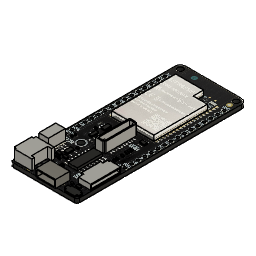
Wemos D32 Pro v13 (Autodesk Fusion 360 design; units mm, degrees)
Autodesk Fusion 360 part; units mm, degrees
sketch "Skizze1" plane through (0, 0, 0) normal (0, 0, 1) x (1, 0, 0)
  line L0 (-12.7, 32.5) -> (12.7, 32.5)
  line L1 (12.7, 32.5) -> (12.7, -32.5)
  line L2 (12.7, -32.5) -> (-12.7, -32.5)
  line L3 (-12.7, -32.5) -> (-12.7, 32.5)
  line L4 (0, 32.5) -> (0, -32.5)
  line L5 (12.7, 0) -> (-12.7, 0)
  line L6 (-8.0924, -22.0419) -> (-2.6557, -22.0419)
  line L7 (-2.6557, -22.0419) -> (-2.6557, -26)
  dimension "d1" = 65
  dimension "d2" = 25.4
  constraint horizontal L0
  constraint vertical L1
  constraint horizontal L2
  constraint vertical L3
  constraint midpoint L0 L4.start
  constraint midpoint L2 L4.end
  constraint coincident origin L4
  constraint midpoint L1 L5.start
  constraint midpoint L3 L5.end
  constraint coincident origin L5
  measures "d1" distance of L0 L2
  measures "d2" distance of L1 L3
extrude "Extrusion1" add sketch "Skizze1" along normal blind 1.57 makes body 1
fillet "Abrundung1" radius 1 2 edges at (12.7, -32.5, 0.785) (-12.7, -32.5, 0.785) on bodies 1
fillet "Abrundung2" radius 2 2 edges at (12.7, 32.5, 0.785) (-12.7, 32.5, 0.785) on bodies 1
sketch "Skizze2" plane through (0, 0, 1.57) normal (0, 0, 1) x (-1, 0, 0)
  arc A0 (10.7, -32.5) -> (12.7, -30.5) centre (10.7, -30.5) ccw
  line L0 (12.7, -30.5) -> (12.7, 31.5)
  arc A1 (12.7, 31.5) -> (11.7, 32.5) centre (11.7, 31.5) ccw
  line L1 (11.7, 32.5) -> (-11.7, 32.5)
  arc A2 (-11.7, 32.5) -> (-12.7, 31.5) centre (-11.7, 31.5) ccw
  line L2 (-12.7, 31.5) -> (-12.7, -30.5)
  arc A3 (-12.7, -30.5) -> (-10.7, -32.5) centre (-10.7, -30.5) ccw
  line L3 (-10.7, -32.5) -> (10.7, -32.5)
  circle A4 centre (5.3, 12.9) radius 1.1365
  circle A5 centre (-11.4, 12.8) radius 0.5
  point P0 (10.7, -30.5)
  point P1 (-10.7, -30.5)
  dimension "d29" = 1
  constraint coincident P0 A0.centre
  constraint coincident P1 A3.centre
  measures "d29" diameter of A5
hole "Bohrung1" at (-10.7, 30.5, 1.57) at (10.7, 30.5, 1.57) direction (0, 0, -1) diameter 2.1 end through all bodies 1
extrude "Extrusion2" cut sketch "Skizze2" against normal through all contours A4 bodies 1
sketch "Skizze3" plane through (0, 0, 1.57) normal (0, 0, 1) x (-1, 0, 0)
  circle A0 centre (5.3, 12.9) radius 1.1365
  circle A1 centre (10.7, -30.5) radius 1.05
  circle A2 centre (-10.7, -30.5) radius 1.05
  arc A3 (10.7, -32.5) -> (12.7, -30.5) centre (10.7, -30.5) ccw
  line L0 (12.7, -30.5) -> (12.7, 31.5)
  arc A4 (12.7, 31.5) -> (11.7, 32.5) centre (11.7, 31.5) ccw
  line L1 (11.7, 32.5) -> (-11.7, 32.5)
  arc A5 (-11.7, 32.5) -> (-12.7, 31.5) centre (-11.7, 31.5) ccw
  line L2 (-12.7, 31.5) -> (-12.7, -30.5)
  arc A6 (-12.7, -30.5) -> (-10.7, -32.5) centre (-10.7, -30.5) ccw
  line L3 (-10.7, -32.5) -> (10.7, -32.5)
  line L4 (8, -26) -> (-8.0924, -26)
  line L5 (-8.0924, -26) -> (-8.0924, -1.543)
  line L6 (-8.0924, -1.543) -> (8, -1.543)
  line L7 (8, -1.543) -> (8, -26)
  line L8 (-8.0924, -22.0419) -> (-2.6557, -22.0419)
  line L9 (-2.6557, -22.0419) -> (-2.6557, -26)
  line L10 (0.3, 12.3) -> (-2.4695, 12.3)
  line L11 (-3.0004, 11.7003) -> (-3.0073, 0.1927)
  line L12 (-3.0073, 0.1927) -> (-2.6232, 0.1927)
  line L13 (-2.6232, 0.1927) -> (-2.6232, -0.5)
  line L14 (-2.6232, -0.5) -> (0.1, -0.5)
  line L15 (0.1, -0.5) -> (0.3, 12.3)
  line L16 (-2.4695, 12.3) -> (-2.4695, 11.7)
  line L17 (-2.4695, 11.7) -> (-3.0004, 11.7003)
  line L18 (12.7, 31.017) -> (12, 31.017)
  line L19 (12, 31.017) -> (12, 31.7213)
  line L20 (12, 31.7213) -> (5.2889, 31.7213)
  line L21 (5.2889, 31.7213) -> (5.2889, 30.6934)
  line L22 (5.2889, 30.6934) -> (6.5, 30.6934)
  line L23 (6.5, 30.6934) -> (6.5, 24.5)
  line L24 (6.5, 24.5) -> (5, 24.5)
  line L25 (5, 24.5) -> (5, 23.5)
  line L26 (5, 23.5) -> (11.9879, 23.5)
  line L27 (11.9879, 23.5) -> (11.9879, 24.4)
  line L28 (11.9879, 24.4) -> (12.7, 24.4)
  line L29 (2.5, 27.5) -> (-5, 27.5)
  line L30 (-5, 27.5) -> (-5, 33)
  line L31 (-5, 33) -> (2.5, 33)
  line L32 (2.5, 33) -> (2.5, 27.5)
  line L33 (-12.284, 15.3134) -> (-8.2222, 15.3134)
  line L34 (-8.2222, 15.3134) -> (-8.2222, 15.7057)
  line L35 (-8.2222, 15.7057) -> (-7.6, 15.7057)
  line L36 (-7.6, 15.7057) -> (-7.6, 17.4)
  line L37 (-7.6, 17.4) -> (-6.7, 17.4)
  line L38 (-6.7, 17.4) -> (-6.7, 24.7236)
  line L39 (-6.7, 24.7236) -> (-7.6, 24.7236)
  line L40 (-7.6, 24.7236) -> (-7.6, 26.8499)
  line L41 (-7.6, 26.8499) -> (-12.2869, 26.8499)
  line L42 (-12.2869, 26.8499) -> (-12.284, 15.3134)
  line L43 (0.2178, 13.2376) -> (-3.3, 13.2376)
  line L44 (-3.3, 13.2376) -> (-3.3, 23)
  line L45 (-3.3, 23) -> (0.2178, 23)
  line L46 (0.2178, 23) -> (0.2178, 13.2376)
  line L47 (-7.6661, 29.4452) -> (-11.5851, 29.4452)
  line L48 (-11.5851, 29.4452) -> (-11.5851, 32.3121)
  line L49 (-11.5851, 32.3121) -> (-7.6661, 32.3121)
  line L50 (-7.6661, 32.3121) -> (-7.6661, 29.4452)
  line L51 (-6.7206, 29.9485) -> (-7.6661, 29.9485)
  line L52 (-7.6661, 29.9485) -> (-7.6661, 31.3971)
  line L53 (-7.6661, 31.3971) -> (-6.7206, 31.3971)
  line L54 (-6.7206, 31.3971) -> (-6.7206, 29.9485)
  line L55 (-11.5851, 30.0095) -> (-12.3019, 30.0095)
  line L56 (-12.3019, 30.0095) -> (-12.3019, 31.3971)
  line L57 (-12.3019, 31.3971) -> (-11.5851, 31.3971)
  line L58 (-11.5851, 31.3971) -> (-11.5851, 30.0095)
  line L59 (-8.3371, 27.7983) -> (-9.9382, 27.7983)
  line L60 (-9.9382, 27.7983) -> (-9.9382, 28.637)
  line L61 (-9.9382, 28.637) -> (-8.3371, 28.637)
  line L62 (-8.3371, 28.637) -> (-8.3371, 27.7983)
  line L63 (-6.2632, 28.0271) -> (-7.1934, 28.0271)
  line L64 (-7.1934, 28.0271) -> (-7.1934, 28.637)
  line L65 (-7.1934, 28.637) -> (-6.2632, 28.637)
  line L66 (-6.2632, 28.637) -> (-6.2632, 28.0271)
  line L67 (1.7274, 24.6112) -> (0.172, 24.6112)
  line L68 (0.172, 24.6112) -> (0.172, 25.4195)
  line L69 (0.172, 25.4195) -> (1.7274, 25.4195)
  line L70 (1.7274, 25.4195) -> (1.7274, 24.6112)
  line L71 (1.7274, 24.1233) -> (0.7057, 24.1233)
  line L72 (0.7057, 24.1233) -> (0.7057, 23.742)
  line L73 (0.7057, 23.742) -> (1.7274, 23.742)
  line L74 (1.7274, 23.742) -> (1.7274, 24.1233)
  line L75 (6.6529, 20.4177) -> (5.0213, 20.4177)
  line L76 (5.0213, 20.4177) -> (5.0213, 21.3174)
  line L77 (5.0213, 21.3174) -> (6.6529, 21.3174)
  line L78 (6.6529, 21.3174) -> (6.6529, 20.4177)
  line L79 (4.1216, 20.4177) -> (2.5356, 20.4177)
  line L80 (2.5356, 20.4177) -> (2.5356, 21.3174)
  line L81 (2.5356, 21.3174) -> (4.1216, 21.3174)
  line L82 (4.1216, 21.3174) -> (4.1216, 20.4177)
  line L83 (7.5, 22) -> (5.5, 22)
  line L84 (5.5, 22) -> (5.5, 23)
  line L85 (5.5, 23) -> (7.5, 23)
  line L86 (7.5, 23) -> (7.5, 22)
  line L87 (4.762, 22.1714) -> (3.6946, 22.1714)
  line L88 (3.6946, 22.1714) -> (3.6946, 22.6441)
  line L89 (3.6946, 22.6441) -> (4.762, 22.6441)
  line L90 (4.762, 22.6441) -> (4.762, 22.1714)
  line L91 (5.4482, 19.3503) -> (3.9996, 19.3503)
  line L92 (3.9996, 19.3503) -> (3.9996, 16.7731)
  line L93 (3.9996, 16.7731) -> (5.4482, 16.7731)
  line L94 (5.4482, 16.7731) -> (5.4482, 19.3503)
  line L95 (4.4113, 15.8429) -> (3.5421, 15.8429)
  line L96 (3.5421, 15.8429) -> (3.5421, 15.2787)
  line L97 (3.5421, 15.2787) -> (4.4113, 15.2787)
  line L98 (4.4113, 15.2787) -> (4.4113, 15.8429)
  line L99 (9.2301, 12.5186) -> (8.6506, 12.5186)
  line L100 (8.6506, 12.5186) -> (8.6506, 13.0066)
  line L101 (8.6506, 13.0066) -> (9.2301, 13.0066)
  line L102 (9.2301, 13.0066) -> (9.2301, 12.5186)
  line L103 (9.2301, 11.2682) -> (8.6506, 11.2682)
  line L104 (8.6506, 11.2682) -> (8.6506, 11.6951)
  line L105 (8.6506, 11.6951) -> (9.2301, 11.6951)
  line L106 (9.2301, 11.6951) -> (9.2301, 11.2682)
  line L107 (3.2371, 6.4952) -> (1.8952, 6.4952)
  line L108 (1.8952, 6.4952) -> (1.8952, 8.8588)
  line L109 (1.8952, 8.8588) -> (3.2371, 8.8588)
  line L110 (3.2371, 8.8588) -> (3.2371, 6.4952)
  line L111 (6.104, 6.4952) -> (4.945, 6.4952)
  line L112 (4.945, 6.4952) -> (4.945, 9.1638)
  line L113 (4.945, 9.1638) -> (6.104, 9.1638)
  line L114 (6.104, 9.1638) -> (6.104, 6.4952)
  line L115 (6.104, 1.9204) -> (4.6553, 1.9204)
  line L116 (4.6553, 1.9204) -> (4.6553, 4.467)
  line L117 (4.6553, 4.467) -> (6.104, 4.467)
  line L118 (6.104, 4.467) -> (6.104, 1.9204)
  line L119 (7.6136, 5.2447) -> (6.5919, 5.2447)
  line L120 (6.5919, 5.2447) -> (6.5919, 5.6717)
  line L121 (6.5919, 5.6717) -> (7.6136, 5.6717)
  line L122 (7.6136, 5.6717) -> (7.6136, 5.2447)
  line L123 (2.6881, 2.0576) -> (1.7274, 2.0576)
  line L124 (1.7274, 2.0576) -> (1.7274, 2.4999)
  line L125 (1.7274, 2.4999) -> (2.6881, 2.4999)
  line L126 (2.6881, 2.4999) -> (2.6881, 2.0576)
  line L127 (3, 1.5) -> (1.4377, 1.5)
  line L128 (1.4377, 1.5) -> (1.4377, 0.8224)
  line L129 (1.4377, 0.8224) -> (3, 0.8224)
  line L130 (3, 0.8224) -> (3, 1.5)
  line L131 (2.7186, 0.182) -> (1.7274, 0.182)
  line L132 (1.7274, 0.182) -> (1.7274, -0.2297)
  line L133 (1.7274, -0.2297) -> (2.7186, -0.2297)
  line L134 (2.7186, -0.2297) -> (2.7186, 0.182)
  line L135 (-6, 0.7) -> (-7.8721, 0.7)
  line L136 (-7.8721, 0.7) -> (-7.8721, 1.9204)
  line L137 (-7.8721, 1.9204) -> (-6, 1.9204)
  line L138 (-6, 1.9204) -> (-6, 0.7)
  line L139 (-6.5262, 5.7061) -> (-7.4932, 5.7061)
  line L140 (-7.4932, 5.7061) -> (-7.4932, 6.1963)
  line L141 (-7.4932, 6.1963) -> (-6.5262, 6.1963)
  line L142 (-6.5262, 6.1963) -> (-6.5262, 5.7061)
  line L143 (-6.5262, 6.5672) -> (-7.4932, 6.5672)
  line L144 (-7.4932, 6.5672) -> (-7.4932, 7.1369)
  line L145 (-7.4932, 7.1369) -> (-6.5262, 7.1369)
  line L146 (-6.5262, 7.1369) -> (-6.5262, 6.5672)
  line L147 (-6.5262, 7.4681) -> (-7.4932, 7.4681)
  line L148 (-7.4932, 7.4681) -> (-7.4932, 8.0245)
  line L149 (-7.4932, 8.0245) -> (-6.5262, 8.0245)
  line L150 (-6.5262, 8.0245) -> (-6.5262, 7.4681)
  line L151 (-6.6984, 9.2963) -> (-7.6522, 9.2963)
  line L152 (-7.6522, 9.2963) -> (-7.6522, 9.8792)
  line L153 (-7.6522, 9.8792) -> (-6.6984, 9.8792)
  line L154 (-6.6984, 9.8792) -> (-6.6984, 9.2963)
  line L155 (-6.6984, 11.3629) -> (-7.6522, 11.3629)
  line L156 (-7.6522, 11.3629) -> (-7.6522, 11.8266)
  line L157 (-7.6522, 11.8266) -> (-6.6984, 11.8266)
  line L158 (-6.6984, 11.8266) -> (-6.6984, 11.3629)
  line L159 (-6.6984, 12.33) -> (-7.6522, 12.33)
  line L160 (-7.6522, 12.33) -> (-7.6522, 12.8069)
  line L161 (-7.6522, 12.8069) -> (-6.6984, 12.8069)
  line L162 (-6.6984, 12.8069) -> (-6.6984, 12.33)
  line L163 (12.7, 15.2249) -> (9.0417, 15.2249)
  line L164 (9.0417, 15.2249) -> (9.0417, 21.6968)
  line L165 (9.0417, 21.6968) -> (12.7, 21.6968)
  line L166 (12.7, 21.6968) -> (12.7, 15.2249)
  constraint horizontal L4
  constraint vertical L5
  constraint horizontal L6
  constraint vertical L7
  constraint coincident L5 L8.start
  constraint perpendicular L5 L8
  constraint coincident L4 L9.end
  constraint perpendicular L4 L9
  constraint horizontal L10
  constraint perpendicular L12 L13
  constraint perpendicular L13 L14
  constraint perpendicular L10 L16
  constraint perpendicular L11 L17
  constraint coincident L0 L18.start
  constraint perpendicular L0 L18
  constraint perpendicular L18 L19
  constraint perpendicular L19 L20
  constraint perpendicular L20 L21
  constraint perpendicular L21 L22
  constraint perpendicular L22 L23
  constraint perpendicular L23 L24
  constraint perpendicular L24 L25
  constraint perpendicular L0 L26
  constraint perpendicular L26 L27
  constraint coincident L0 L28.end
  constraint perpendicular L0 L28
  constraint perpendicular L0 L29
  constraint perpendicular L1 L30
  constraint perpendicular L0 L31
  constraint perpendicular L29 L32
  constraint perpendicular L2 L33
  constraint perpendicular L33 L34
  constraint perpendicular L2 L35
  constraint perpendicular L33 L36
  constraint perpendicular L2 L37
  constraint perpendicular L33 L38
  constraint perpendicular L38 L39
  constraint perpendicular L33 L40
  constraint perpendicular L40 L41
  constraint horizontal L43
  constraint vertical L44
  constraint horizontal L45
  constraint vertical L46
  constraint horizontal L47
  constraint vertical L48
  constraint horizontal L49
  constraint vertical L50
  constraint horizontal L51
  constraint vertical L52
  constraint horizontal L53
  constraint vertical L54
  constraint coincident L50 L52.end
  constraint horizontal L55
  constraint vertical L56
  constraint horizontal L57
  constraint vertical L58
  constraint coincident L48 L55.start
  constraint horizontal L59
  constraint vertical L60
  constraint horizontal L61
  constraint vertical L62
  constraint horizontal L63
  constraint vertical L64
  constraint horizontal L65
  constraint vertical L66
  constraint horizontal L67
  constraint vertical L68
  constraint horizontal L69
  constraint vertical L70
  constraint horizontal L71
  constraint vertical L72
  constraint horizontal L73
  constraint vertical L74
  constraint horizontal L75
  constraint vertical L76
  constraint horizontal L77
  constraint vertical L78
  constraint horizontal L79
  constraint vertical L80
  constraint horizontal L81
  constraint vertical L82
  constraint horizontal L83
  constraint vertical L84
  constraint horizontal L85
  constraint vertical L86
  constraint horizontal L87
  constraint vertical L88
  constraint horizontal L89
  constraint vertical L90
  constraint horizontal L91
  constraint vertical L92
  constraint horizontal L93
  constraint vertical L94
  constraint horizontal L95
  constraint vertical L96
  constraint horizontal L97
  constraint vertical L98
  constraint horizontal L99
  constraint vertical L100
  constraint horizontal L101
  constraint vertical L102
  constraint horizontal L103
  constraint vertical L104
  constraint horizontal L105
  constraint vertical L106
  constraint horizontal L107
  constraint vertical L108
  constraint horizontal L109
  constraint vertical L110
  constraint horizontal L111
  constraint vertical L112
  constraint horizontal L113
  constraint vertical L114
  constraint horizontal L115
  constraint vertical L116
  constraint horizontal L117
  constraint vertical L118
  constraint horizontal L119
  constraint vertical L120
  constraint horizontal L121
  constraint vertical L122
  constraint horizontal L123
  constraint vertical L124
  constraint horizontal L125
  constraint vertical L126
  constraint horizontal L127
  constraint vertical L128
  constraint horizontal L129
  constraint vertical L130
  constraint horizontal L131
  constraint vertical L132
  constraint horizontal L133
  constraint vertical L134
  constraint horizontal L135
  constraint vertical L136
  constraint horizontal L137
  constraint vertical L138
  constraint horizontal L139
  constraint vertical L140
  constraint horizontal L141
  constraint vertical L142
  constraint horizontal L143
  constraint vertical L144
  constraint horizontal L145
  constraint vertical L146
  constraint horizontal L147
  constraint vertical L148
  constraint horizontal L149
  constraint vertical L150
  constraint horizontal L151
  constraint vertical L152
  constraint horizontal L153
  constraint vertical L154
  constraint horizontal L155
  constraint vertical L156
  constraint horizontal L157
  constraint vertical L158
  constraint horizontal L159
  constraint vertical L160
  constraint horizontal L161
  constraint vertical L162
  constraint horizontal L163
  constraint vertical L164
  constraint horizontal L165
  constraint vertical L166
  constraint coincident L0 L163.start
extrude "Extrusion3" add sketch "Skizze3" along normal blind 2 separate body contours L4 L5 L6 L7 L8 L9 makes body 2
extrude "Extrusion4" add sketch "Skizze3" along normal blind 1 contours L43 L44 L45 L46 bodies 2 1
extrude "Extrusion5" add sketch "Skizze3" along normal blind 0.5 contours L47 L48 L49 L50 L52 L58 | L50 L51 L52 L53 L54 | L48 L55 L56 L57 L58 | L59 L60 L61 L62 | L63 L64 L65 L66 | L67 L68 L69 L70 | L71 L72 L73 L74 | L75 L76 L77 L78 | L79 L80 L81 L82 | L83 L84 L85 L86 | L87 L88 L89 L90 | L91 L92 L93 L94 | L95 L96 L97 L98 | L99 L100 L101 L102 | L103 L104 L105 L106 | L107 L108 L109 L110 | L111 L112 L113 L114 | L115 L116 L117 L118 | L119 L120 L121 L122 | L123 L124 L125 L126 | L127 L128 L129 L130 | L131 L132 L133 L134 | L135 L136 L137 L138 | L139 L140 L141 L142 | L143 L144 L145 L146 | L147 L148 L149 L150 | L151 L152 L153 L154 | L155 L156 L157 L158 | L159 L160 L161 L162 bodies 1
extrude "Extrusion6" add sketch "Skizze3" along normal blind 4 separate body contours L10 L11 L12 L13 L14 L15 L16 L17 makes body 3
extrude "Extrusion7" add sketch "Skizze3" along normal blind 3 separate body contours L1 L30 L31 L32 | L1 L29 L30 L32 makes body 4
extrude "Extrusion8" add sketch "Skizze3" along normal blind 4 separate body contours L0 L163 L164 L165 L166 | L0 L18 L19 L20 L21 L22 L23 L24 L25 L26 L27 L28 makes body 5 at (-10.1626, -28.7035, 1.57) makes body 6 at (-12.7, -17.3822, 2.9033)
extrude "Extrusion9" add sketch "Skizze3" along normal blind 2 separate body contours L33 L34 L35 L36 L37 L38 L39 L40 L41 L42 makes body 7
shell "Schale1" thickness 0.5 removed faces 1 at (0.7411, -3.9976, 5.57) on bodies 3
shell "Schale2" thickness 0.4 removed faces 4 at (2.5, -33, 2.57) at (-12.7, -26.6057, 2.9033) at (-12.7, -17.3822, 2.9033) at (12.286, -23.0044, 2.2367) on bodies 4 5 6 7
extrude "Extrusion10" cut sketch "Skizze2" against normal through all contours A5 bodies 1
pattern_linear "R-Anordnung1" count 16 spacing 2.5333 along (0, 1, 0) of "Extrusion10"
mirror "Spiegeln1" about plane through (0, 0, 0) normal (1, 0, 0) of "Extrusion10", "R-Anordnung1"
copy_body "Körper->Berechn1" bodies 1 removing the originals makes body 8 in component "Component"
copy_body "Körper->Berechn2" bodies 6 removing the originals makes body 9 in component "Component'"
copy_body "Körper->Berechn3" bodies 4 removing the originals makes body 10 in component "Component''"
copy_body "Körper->Berechn4" bodies 5 removing the originals makes body 11 in component "Component'''"
copy_body "Körper->Berechn5" bodies 3 removing the originals makes body 12 in component "Component''''"
copy_body "Körper->Berechn6" bodies 7 removing the originals makes body 13 in component "Component'''''"
copy_body "Körper->Berechn7" bodies 2 removing the originals makes body 14 in component "Component''''''"
component "Component" placed x (1, 0, 0) y (0, 1, 0) z (0, 0, 1) at (0, 0, 0)
component "Component'" placed x (1, 0, 0) y (0, 1, 0) z (0, 0, 1) at (0, 0, 0)
component "Component''" placed x (1, 0, 0) y (0, 1, 0) z (0, 0, 1) at (0, 0, 0)
component "Component'''" placed x (1, 0, 0) y (0, 1, 0) z (0, 0, 1) at (0, 0, 0)
component "Component''''" placed x (1, 0, 0) y (0, 1, 0) z (0, 0, 1) at (0, 0, 0)
component "Component'''''" placed x (1, 0, 0) y (0, 1, 0) z (0, 0, 1) at (0, 0, 0)
component "Component''''''" placed x (1, 0, 0) y (0, 1, 0) z (0, 0, 1) at (0, 0, 0)
